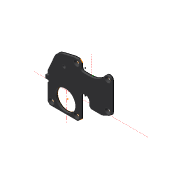
# Autodesk Inventor part: COXA_YAW_ROLL_ADPT_TOP_BASE
Saved by Autodesk Inventor 2019.4 (Build 234330000, 330)
## iProperties
Created: 2019-11-06
Part Number: COXA_YAW_ROLL_ADPT_TOP_BASE
Material: 一般
Document SubType Name: Modeling
Designer: y6tada
Density: 1 g/cm^3
Appearance: Black 100
Author: y6tada
Autodesk Inventor part; units mm, degrees
ref_plane "YZ Plane" through (0, 0, 0) normal (1, 0, 0) x (0, 1, 0)
ref_plane "XZ Plane" through (0, 0, 0) normal (0, 1, 0) x (-1, 0, 0)
ref_plane "XY Plane" through (0, 0, 0) normal (0, 0, 1) x (1, 0, 0)
sketch "スケッチ1" plane through (0, 0, 0) normal (0, 0, 1) x (1, 0, 0)
  circle A0 centre (11, -20) radius 1.25 construction
  circle A1 centre (11, 20) radius 1.25 construction
  circle A2 centre (-11, -20) radius 1.25 construction
  arc A3 (8.5, 20) -> (11, 17.5) centre (11, 20) ccw construction
  line L0 (11, 17.5) -> (12.15, 17.5) construction
  arc A4 (13.15, 16.5) -> (12.15, 17.5) centre (12.15, 16.5) ccw construction
  line L1 (13.15, 16.5) -> (13.15, -16.5) construction
  arc A5 (12.15, -17.5) -> (13.15, -16.5) centre (12.15, -16.5) ccw construction
  line L2 (12.15, -17.5) -> (11, -17.5) construction
  arc A6 (11, -17.5) -> (8.5, -20) centre (11, -20) ccw construction
  line L3 (8.5, -20) -> (8.5, -21.15) construction
  arc A7 (7.5, -22.15) -> (8.5, -21.15) centre (7.5, -21.15) ccw construction
  line L4 (7.5, -22.15) -> (-7.5, -22.15) construction
  arc A8 (-8.5, -21.15) -> (-7.5, -22.15) centre (-7.5, -21.15) ccw construction
  line L5 (-8.5, -21.15) -> (-8.5, -20) construction
  arc A9 (-8.5, -20) -> (-11, -17.5) centre (-11, -20) ccw construction
  line L6 (-11, -17.5) -> (-14, -17.5) construction
  line L7 (8.5, 23) -> (8.5, 20) construction
  line L8 (-14.25, -17.75) -> (-14.25, -21.25) construction
  line L9 (-14.25, -21.25) -> (-12.25, -23.25) projected
  line L10 (-12.25, -23.25) -> (12.25, -23.25) projected
  line L11 (12.25, -23.25) -> (14.25, -21.25) projected
  line L12 (14.25, -21.25) -> (14.25, 21.25) construction
  line L13 (14.25, 21.25) -> (12.25, 23.25) projected
  line L14 (12.25, 23.25) -> (8.75, 23.25) construction
  line L15 (16.75, 15.618) -> (22.25, 15.618)
  line L16 (41.3, 21.118) -> (41.3, -2.882)
  line L17 (19.75, -0.382) -> (16.75, -0.382)
  arc A10 (41.3, 21.118) -> (35.8184, 22.8038) centre (38.3, 21.118) ccw
  arc A11 (39.5165, -5.6243) -> (41.3, -2.882) centre (38.3, -2.882) ccw
  circle A12 centre (38.3, 21.118) radius 1.25 construction
  circle A13 centre (38.3, -2.882) radius 1.25 construction
  line L18 (14.25, 21.25) -> (14.25, 18.118)
  line L19 (14.25, -2.882) -> (14.25, -21.25)
  arc A14 (14.25, 18.118) -> (16.75, 15.618) centre (16.75, 18.118) ccw
  arc A15 (16.75, -0.382) -> (14.25, -2.882) centre (16.75, -2.882) ccw
  line L20 (72.306, -6.882) -> (-28.676, -6.882) construction
  circle A16 centre (1.21, -13.01) radius 8.7 construction
  circle A17 centre (1.21, -13.01) radius 8.95
  arc A18 (22.25, 15.618) -> (35.8184, 22.8038) centre (22.25, 32.0211) ccw
  line L21 (22.25, 32.0211) -> (22.25, -5.382) construction
  line L22 (22.25, -2.882) -> (22.25, -5.882)
  line L23 (24.75, -8.382) -> (33.3, -8.382)
  line L24 (33.3, -8.382) -> (39.5165, -5.6243)
  arc A19 (22.25, -2.882) -> (19.75, -0.382) centre (19.75, -2.882) ccw
  arc A20 (22.25, -5.882) -> (24.75, -8.382) centre (24.75, -5.882) ccw
  circle A21 centre (0, 12) radius 1.25 construction
  line L25 (12.25, 23.25) -> (8.5, 23.25)
  line L26 (8.5, 23.25) -> (-2.0647, 20.76)
  arc A22 (-2.0647, 20.76) -> (-8.234, 15.6334) centre (0, 12) ccw
  line L27 (0, 0) -> (0, -31.805) construction
  line L28 (-12.15, -17.5) -> (-14.25, -17.5) construction
  line L29 (8.5, 23.25) -> (8.5, 21.15) construction
  line L30 (8.75, 23.25) -> (8.5, 23) projected
  line L31 (-14, -17.5) -> (-14.25, -17.75) construction
  line L32 (-14.25, 0) -> (-14.25, -2) construction
  line L33 (-14.25, -2) -> (-16.25, -2)
  line L34 (-16.25, -2) -> (-16.25, -5)
  line L35 (-16.25, -5) -> (-14.25, -5)
  line L36 (-14.25, -5) -> (-14.25, -7) construction
  line L37 (-14.25, 0) -> (-14.25, 2)
  line L38 (-14.25, 2) -> (-8.234, 15.6334)
  arc A23 (-14.25, -2) -> (-14.25, 0) centre (-14.25, -1) ccw
  arc A24 (-14.25, -7) -> (-14.25, -5) centre (-14.25, -6) ccw
  line L39 (-14.25, -7) -> (-14.25, -21.25)
  point P0 (11, 20)
  point P1 (11, -20)
  point P2 (-11, -20)
  point P3 (14.25, 15.618)
  point P4 (23.6679, 15.618)
  point P5 (23.161, -0.382)
  point P6 (14.25, -0.382)
  point P7 (22.25, -0.382)
  dimension "d0" = 3
  dimension "d1" = 2.5
  dimension "d2" = 6.5
  dimension "d3" = 0.25
  dimension "d7" = 16
  dimension "d8" = 8
  dimension "d16" = 8
  dimension "d17" = 5
  dimension "d26" = 9
  dimension "d34" = 1
  dimension "d35" = 3
  dimension "d36" = 2
  dimension "d37" = 10
  dimension "d38" = 2
  constraints: 46 end point, 20 point on circle, 17 tangent, 14 point on line, 11 centre point, 8 vertical, 6 coincident, 5 equal radius, 5 perpendicular, 3 concentric, 3 horizontal, 2 collinear, 2 other
  measures "d0" radius of A10
  measures "d1" radius of A14
  measures "d2" distance between parallel lines of L20 L17
  measures "d3" radial gap between concentric circles of A16 A17
  measures "d7" distance between parallel lines of L17 L15
  measures "d8" distance between parallel lines of L12 L21
  measures "d16" distance between parallel lines of L17 L23
  measures "d17" horizontal distance of L23.end point (38.3, -2.882)
  measures "d26" radius of A22
  measures "d34" radius of A24
  measures "d35" distance of L33.end L34.end
  measures "d36" distance of L32.start L37.end
  measures "d37" vertical distance of point (0, 12) L37.end
  measures "d38" distance between parallel lines of L32 L34
extrude "押し出し1" add sketch "スケッチ1" along normal blind 2
sketch "スケッチ2" plane through (0, 0, 2) normal (0, 0, 1) x (1, 0, 0)
  point P0 (0, 0)
  point P1 (38.3, 21.118)
  point P2 (38.3, -2.882)
  point P3 (-11, 20)
  point P4 (11, 20)
  point P5 (11, -20)
  point P6 (-11, -20)
hole "穴2" at (38.3, 21.118, 2) at (38.3, -2.882, 2) at (-11, 20, 2) at (11, 20, 2) at (11, -20, 2) at (-11, -20, 2) direction (0, 0, -1) diameter 2.5 end through all countersink diameter 5 countersink angle 90
hole "穴3" at (0, 12, 0) direction (0, 0, 1) diameter 3 end through all
chamfer "面取り1" distance 0.25 angle 45 2 edges at (-16.25, -2, 1) (-16.25, -5, 1)
